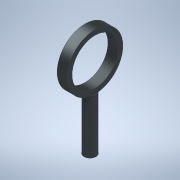
# Autodesk Inventor part: hook
Saved by Autodesk Inventor 2021.5 (Build 255421000, 421)
## iProperties
Created: 2024-11-18
Part Number: hook
Material: Iron, Cast
Document SubType Name: Modeling
Designer: email
Density: 7.15 g/cm^3
Appearance: Iron Gray
Author: email
Autodesk Inventor part; units mm, degrees
ref_plane "YZ Plane" through (0, 0, 0) normal (1, 0, 0) x (0, 1, 0)
ref_plane "XZ Plane" through (0, 0, 0) normal (0, 1, 0) x (-1, 0, 0)
ref_plane "XY Plane" through (0, 0, 0) normal (0, 0, 1) x (1, 0, 0)
sketch "Sketch1" plane through (0, 0, 0) normal (0, 1, 0) x (-1, 0, 0)
  circle A0 centre (0, 0) radius 3
  dimension "d0" = 6
  constraints: 1 centre point, 1 coincident
  measures "d0" diameter of A0
extrude "Extrusion1" add sketch "Sketch1" along normal blind 27
sketch "Sketch2" plane through (0, 0, 0) normal (1, 0, 0) x (0, 1, 0)
  line L0 (27, -3) -> (27, 3) projected
  line L1 (27, 0) -> (32.8849, 0)
  circle A0 centre (41, 0) radius 14
  circle A1 centre (41, 0) radius 11.5
  point P0 (0, 0)
  dimension "d4" = 28
  dimension "d7" = 23
  constraints: 2 centre point, 2 end point, 1 coincident, 1 horizontal, 1 midpoint, 1 tangent
  measures "d4" diameter of A0
  measures "d7" diameter of A1
extrude "Extrusion2" add sketch "Sketch2" along normal mid plane 5
body "Solid1"
